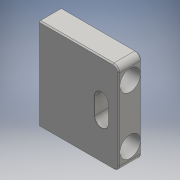
# Autodesk Inventor part: ОПОРА_01
Saved by Autodesk Inventor 2016 (Build 200138000, 138)
## iProperties
Created: 2021-05-03
Part Number: ОПОРА_01
Material: Типовые
Document SubType Name: Modeling
Designer: Лол
Density: 1 g/cm^3
Appearance: По умолчанию
Author: Лол
Autodesk Inventor part; units mm, degrees
ref_plane "YZ Plane" through (0, 0, 0) normal (1, 0, 0) x (0, 1, 0)
ref_plane "XZ Plane" through (0, 0, 0) normal (0, 1, 0) x (-1, 0, 0)
ref_plane "XY Plane" through (0, 0, 0) normal (0, 0, 1) x (1, 0, 0)
sketch "Эскиз1" plane through (0, 0, 0) normal (1, 0, 0) x (0, 1, 0)
  line L0 (-14, 0) -> (14, 0) projected
  line L1 (0, -56) -> (0, 56) projected
  line L2 (10, 40) -> (-10, 40)
  line L3 (-10, 40) -> (-10, -40)
  line L4 (-10, -40) -> (10, -40)
  line L5 (10, -40) -> (10, 40)
  point P0 (0, 0)
  dimension "d0" = 20
  dimension "d1" = 10
  dimension "d2" = 80
  dimension "d3" = 40
  constraints: 8 end point, 2 parallel, 1 horizontal, 1 perpendicular
  measures "d0" distance of L3.end L4.end
  measures "d1" distance between parallel lines of L5 L1
  measures "d2" distance of L2.end L3.end
  measures "d3" distance between parallel lines of L4 L0
extrude "Выдавливание1" add sketch "Эскиз1" against normal blind 70
sketch "Эскиз2" plane through (0, 0, 0) normal (1, 0, 0) x (0, 1, 0)
  line L0 (0, 56) -> (0, -56) projected
  line L1 (0, -56) -> (0, 56) projected
  line L2 (-14, 0) -> (14, 0) projected
  circle A0 centre (0, 25) radius 5
  circle A1 centre (0, -25) radius 5
  line L3 (10, 40) -> (-10, 40) projected
  line L4 (-10, -40) -> (10, -40) projected
  point P0 (0, 0)
  dimension "d6" = 10
  dimension "d7" = 10
  dimension "d10" = 15
  dimension "d12" = 15
  constraints: 2 centre point, 2 point on line
  measures "d6" diameter of A1
  measures "d7" diameter of A0
  measures "d10" distance from line of L3 A0.centre
  measures "d12" distance from line of A1.centre L4
hole "Отверстие1" at (0, 0, 25) at (0, 0, -25) direction (-1, 0, 0) diameter 10.5 end through all counterbore diameter 18 counterbore depth 13.5
fillet "Сопряжение1" radius 5 2 edges at (0, 0, 40) (0, 0, -40)
chamfer "Фаска1" distance 1 angle 45 10 edges at (-37.5, 10, 40) (-1.4645, 10, 38.5355) (0, 10, 0) (-1.4645, 10, -38.5355) (-37.5, 10, -40) (-37.5, -10, 40) (-1.4645, -10, 38.5355) (0, -10, 0) (-1.4645, -10, -38.5355) (-37.5, -10, -40)
chamfer "Фаска2" distance 1 angle 45 4 edges at (-70, 10, 0) (-70, 0, 40) (-70, -10, 0) (-70, 0, -40)
sketch "Эскиз3" plane through (-70, 0, 0) normal (-1, 0, 0) x (0, 0, 1)
  line L0 (-56, 0) -> (56, 0) projected
  line L1 (0, 14) -> (0, -14) projected
  line L2 (-56, 0) -> (56, 0) projected
  circle A0 centre (-14, 0) radius 3
  circle A1 centre (14, 0) radius 3
  circle A2 centre (-25, 0) radius 5.25 projected
  circle A3 centre (25, 0) radius 5.25 projected
  point P0 (0, 0)
  dimension "d28" = 6
  dimension "d29" = 11
  dimension "d30" = 28
  constraints: 2 centre point, 2 point on line, 1 equal radius
  measures "d28" diameter of A0
  measures "d29" distance of A0.centre A2.centre
  measures "d30" distance of A1.centre A0.centre
hole "Отверстие2" at (-70, 0, -14) at (-70, 0, 14) direction (1, 0, 0) diameter 6 depth 10 tip angle 118 countersink diameter 8 countersink angle 45
chamfer "Фаска3" distance 0.4 angle 45 2 edges at (-70, 0, -19.75) (-70, 0, 30.25)
sketch "Эскиз4" plane through (0, 0, 0) normal (0, 1, 0) x (-1, 0, 0)
  line L0 (69.6, 19.75) -> (13.5, 19.75) projected
  line L1 (69.6, -19.75) -> (13.5, -19.75) projected
  line L2 (70, -39) -> (70, 39) projected
  arc A0 (21, 7.5) -> (9, 7.5) centre (15, 7.5) ccw
  arc A1 (9, -7.5) -> (21, -7.5) centre (15, -7.5) ccw
  line L3 (15, 7.5) -> (15, -7.5) construction
  line L4 (-14, 0) -> (84, 0) projected
  line L5 (0, -56) -> (0, 56) projected
  line L6 (0, 25) -> (0, 25) projected
  line L7 (0, 25) -> (0, 25) projected
  line L8 (13.5, 34) -> (13.5, 16) projected
  line L9 (21, 7.5) -> (21, -7.5)
  line L10 (9, 7.5) -> (9, -7.5)
  point P0 (0, 0)
  dimension "d41" = 12
  dimension "d42" = 15
  dimension "d43" = 7.5
  dimension "d44" = 55
  constraints: 6 end point, 4 point on circle, 3 tangent, 2 centre point, 2 vertical, 1 coincident, 1 equal radius
  measures "d41" diameter of A0
  measures "d42" distance of A1.centre L3.start
  measures "d43" distance from line of L3.start L4
  measures "d44" distance between parallel lines of L2 L3
extrude "Выдавливание2" cut sketch "Эскиз4" along normal through all both and the other way through all
chamfer "Фаска4" distance 0.2 angle 45 8 edges at (-15, -10, 13.5) (-9, -10, 0) (-15, -10, -13.5) (-21, -10, 0) (-21, 10, 0) (-15, 10, -13.5) (-9, 10, 0) (-15, 10, 13.5)
